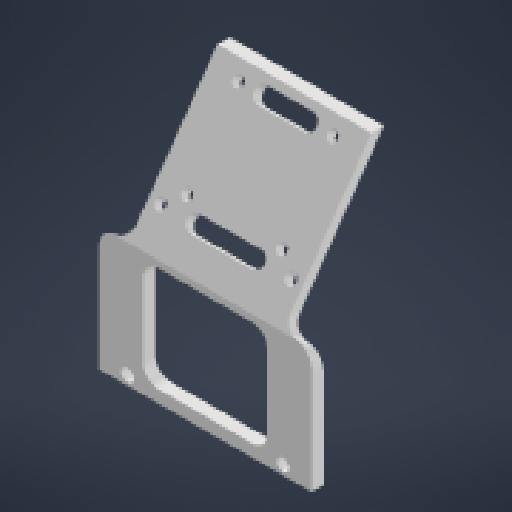
# Autodesk Inventor part: UserInterface mount
Saved by Autodesk Inventor 2023 (Build 270158000, 158)
## iProperties
Created: 2024-01-05
Part Number: UserInterface mount
Material: Generic
Document SubType Name: Modeling
Designer: nick_
Density: 1 g/cm^3
Appearance: Default
Author: nick_
Autodesk Inventor part; units mm, degrees
ref_plane "YZ Plane" through (0, 0, 0) normal (1, 0, 0) x (0, 1, 0)
ref_plane "XZ Plane" through (0, 0, 0) normal (0, 1, 0) x (-1, 0, 0)
ref_plane "XY Plane" through (0, 0, 0) normal (0, 0, 1) x (1, 0, 0)
sketch "Sketch1" plane through (0, 0, 0) normal (0, 0, 1) x (1, 0, 0)
  circle A0 centre (42.125, -15.4) radius 2 construction
  circle A1 centre (-7.875, -15.4) radius 2 construction
  line L0 (-4.825, -12.4) -> (-2.825, -14.4) construction
  line L1 (-9.825, -12.4) -> (-4.825, -12.4) construction
  arc A2 (-14.825, -7.4) -> (-9.825, -12.4) centre (-9.825, -7.4) ccw construction
  line L2 (-14.825, -7.4) -> (-14.825, 13.6) construction
  line L3 (-14.825, 13.6) -> (-15.625, 13.6) construction
  line L4 (-15.625, 13.6) -> (-15.625, 14.6) construction
  line L5 (-14.825, 15.4) -> (-15.625, 14.6) construction
  line L6 (-14.825, 15.4) -> (-14.825, 18.4) construction
  line L7 (-14.825, 18.4) -> (-17.125, 18.4) construction
  line L8 (-17.125, 18.4) -> (-17.125, -18.4) construction
  line L9 (-17.125, -18.4) -> (51.375, -18.4) construction
  line L10 (51.375, 18.4) -> (51.375, -18.4) construction
  line L11 (49.075, 18.4) -> (51.375, 18.4) construction
  line L12 (49.075, 15.4) -> (49.075, 18.4) construction
  line L13 (49.875, 14.6) -> (49.075, 15.4) construction
  line L14 (49.875, 13.6) -> (49.875, 14.6) construction
  line L15 (49.075, 13.6) -> (49.875, 13.6) construction
  line L16 (49.075, -7.4) -> (49.075, 13.6) construction
  arc A3 (44.075, -12.4) -> (49.075, -7.4) centre (44.075, -7.4) ccw construction
  line L17 (39.075, -12.4) -> (44.075, -12.4) construction
  line L18 (37.075, -14.4) -> (39.075, -12.4) construction
  line L19 (37.075, -14.4) -> (-2.825, -14.4) construction
  line L20 (-17.125, -18.4) -> (51.375, -18.4)
  line L21 (51.375, -18.4) -> (51.375, 21.449)
  line L22 (51.375, 21.449) -> (-17.125, 21.449)
  line L23 (-17.125, 21.449) -> (-17.125, -18.4)
  point P0 (0, 0)
  constraints: 8 end point, 2 collinear, 1 perpendicular, 1 point on line
extrude "Extrusion1" add sketch "Sketch1" along normal blind 4
sketch "Sketch2" plane through (51.375, -18.4, 0) normal (1, 0, 0) x (0, 0, -1)
  line L0 (0, 0) -> (0, 39.849) construction
  line L1 (0, 39.849) -> (-4, 39.849) construction
  line L2 (-4, 0) -> (-4, 39.849) construction
  line L3 (0, 0) -> (-4, 0) construction
  line L4 (-4, 39.849) -> (24.6788, 80.8066)
  line L5 (24.6788, 80.8066) -> (28.6788, 80.8066)
  line L6 (28.6788, 80.8066) -> (0, 39.849)
  line L7 (-4, 39.849) -> (0, 39.849)
  point P0 (0, 18.4)
  dimension "d2" = 55
  dimension "d5" = 50
  constraints: 8 end point, 2 equal length, 1 horizontal
  measures "d2" angle of L1 L4
  measures "d5" distance of L1.end L4.end
extrude "Extrusion2" add sketch "Sketch2" against normal up to surface (68.5 mm away)
sketch "Sketch4" plane through (-17.125, 21.449, 4) normal (0, 0.5735764, 0.819152) x (1, 0, 0)
  line L0 (22.585, 45) -> (45.915, 45) construction
  line L1 (45.915, 45) -> (45.915, 22.57) construction
  line L2 (45.915, 22.57) -> (22.585, 22.57) construction
  line L3 (22.585, 22.57) -> (22.585, 45) construction
  line L4 (68.5, 50) -> (0, 50) construction
  point P0 (17.125, -15.2757)
  point P1 (34.25, 45)
  point P2 (34.25, 50)
  dimension "d11" = 23.33
  dimension "d12" = 22.43
  dimension "d13" = 5
  constraints: 8 end point, 4 coincident, 2 midpoint, 2 parallel, 1 horizontal, 1 perpendicular, 1 vertical alignment
  measures "d11" distance of L0.start L0.end
  measures "d12" distance of L0.end L1.end
  measures "d13" distance between parallel lines of L4 L0
hole "Hole1" at (5.46, 58.3109, -21.8109) at (28.79, 58.3109, -21.8109) at (28.79, 39.9373, -8.9456) at (5.46, 39.9373, -8.9456) direction (0, -0.5735764, -0.819152) diameter 3.5 end through all
sketch "Sketch5" plane through (-17.125, 21.449, 4) normal (0, 0.5735764, 0.819152) x (1, 0, 0)
  circle A0 centre (45.915, 22.57) radius 1.75 projected
  circle A1 centre (22.585, 45) radius 1.75 projected
  circle A2 centre (45.915, 45) radius 1.75 projected
  circle A3 centre (22.585, 22.57) radius 1.75 projected
  line L0 (0, 50) -> (0, 0) projected
  line L1 (68.5, 0) -> (0, 0) projected
  line L2 (68.5, 50) -> (68.5, 0) projected
  line L3 (68.5, 50) -> (0, 50) projected
  line L4 (28.75, 45) -> (39.75, 45) construction
  line L5 (28.75, 47.5) -> (39.75, 47.5)
  line L6 (39.75, 42.5) -> (28.75, 42.5)
  arc A4 (28.75, 47.5) -> (28.75, 42.5) centre (28.75, 45) ccw
  arc A5 (39.75, 42.5) -> (39.75, 47.5) centre (39.75, 45) ccw
  point P0 (17.125, -15.2757)
  point P1 (34.25, 45)
  dimension "d25" = 23.33
  dimension "d26" = 5
  dimension "d27" = 11
  dimension "d28" = 11.665
  constraints: 8 end point, 4 point on circle, 4 tangent, 2 centre point, 1 horizontal, 1 horizontal alignment, 1 midpoint, 1 parallel
  measures "d25" distance of A2.centre A1.centre
  measures "d26" distance between parallel lines of L6 L5
  measures "d27" distance of L4.start L4.end
  measures "d28" distance of A1.centre point (34.25, 45)
extrude "Extrusion3" cut sketch "Sketch5" against normal through all contours L5 A5 L6 A4
sketch "Sketch6" plane through (-17.125, 21.449, 4) normal (0, 0.5735764, 0.819152) x (1, 0, 0)
  line L0 (24.25, 17.57) -> (44.25, 17.57) construction
  line L1 (24.25, 15.07) -> (44.25, 15.07)
  line L2 (44.25, 20.07) -> (24.25, 20.07)
  arc A0 (24.25, 20.07) -> (24.25, 15.07) centre (24.25, 17.57) ccw
  arc A1 (44.25, 15.07) -> (44.25, 20.07) centre (44.25, 17.57) ccw
  line L3 (68.5, 0) -> (0, 0) projected
  circle A2 centre (22.585, 22.57) radius 1.75 projected
  point P0 (17.125, -15.2757)
  point P1 (34.25, 17.57)
  point P2 (34.25, 0)
  dimension "d31" = 5
  dimension "d32" = 20
  dimension "d33" = 5
  constraints: 8 end point, 4 point on circle, 4 tangent, 2 centre point, 2 midpoint, 1 horizontal, 1 parallel, 1 vertical alignment
  measures "d31" distance between parallel lines of L1 L2
  measures "d32" distance of L0.start L0.end
  measures "d33" distance from line of L0 A2.centre
extrude "Extrusion4" cut sketch "Sketch6" against normal through all contours A0 L2 A1 L1
sketch "Sketch7" plane through (-17.125, 21.449, 4) normal (0, 0.5735764, 0.819152) x (1, 0, 0)
  line L0 (24.25, 20.07) -> (44.25, 20.07) projected
  line L1 (68.5, 0) -> (0, 0) projected
  point P0 (17.125, -15.2757)
  point P1 (13.25, 11.5)
  point P2 (55.25, 11.5)
  point P3 (34.25, 20.07)
  dimension "d36" = 42
  dimension "d37" = 21
  dimension "d45" = 11.5
  constraints: 1 horizontal alignment, 1 midpoint
  measures "d36" distance of point (55.25, 11.5) point (13.25, 11.5)
  measures "d37" horizontal distance of point (34.25, 20.07) point (13.25, 11.5)
  measures "d45" distance from line of L1 point (55.25, 11.5)
hole "Hole2" at (-3.875, 30.8693, -2.5961) at (38.125, 30.8693, -2.5961) direction (0, -0.5735764, -0.819152) diameter 3.5 end through all
sketch "Sketch8" plane through (-17.125, 21.449, 4) normal (0, 0.5735764, 0.819152) x (1, 0, 0)
  line L0 (0, 25.2888) -> (68.5, 25.2888) construction
  circle A0 centre (13.25, 11.5) radius 1.75 construction
  circle A1 centre (55.25, 11.5) radius 1.75 construction
  line L1 (24.25, 20.07) -> (44.25, 20.07) construction
  arc A2 (44.25, 15.07) -> (44.25, 20.07) centre (44.25, 17.57) ccw construction
  line L2 (44.25, 15.07) -> (24.25, 15.07) construction
  arc A3 (24.25, 20.07) -> (24.25, 15.07) centre (24.25, 17.57) ccw construction
  arc A4 (28.75, 47.5) -> (28.75, 42.5) centre (28.75, 45) ccw construction
  line L3 (28.75, 47.5) -> (39.75, 47.5) construction
  arc A5 (39.75, 42.5) -> (39.75, 47.5) centre (39.75, 45) ccw construction
  line L4 (39.75, 42.5) -> (28.75, 42.5) construction
  circle A6 centre (45.915, 22.57) radius 1.75 construction
  circle A7 centre (22.585, 45) radius 1.75 construction
  circle A8 centre (45.915, 45) radius 1.75 construction
  circle A9 centre (22.585, 22.57) radius 1.75 construction
  line L5 (0, 50) -> (0, 0) construction
  line L6 (68.5, 0) -> (0, 0) construction
  line L7 (68.5, 50) -> (68.5, 0) construction
  line L8 (68.5, 50) -> (0, 50) construction
  line L9 (0, 0) -> (9.5, 0)
  line L10 (9.5, 0) -> (9.5, 54)
  line L11 (9.5, 54) -> (0, 54)
  line L12 (0, 54) -> (0, 0)
  line L13 (68.5, 0) -> (59, 0)
  line L14 (59, 0) -> (59, 54)
  line L15 (59, 54) -> (68.5, 54)
  line L16 (68.5, 54) -> (68.5, 0)
  point P0 (17.125, -15.2757)
  dimension "d50" = 9.5
  dimension "d51" = 9.5
  dimension "d52" = 4
  constraints: 16 end point, 4 parallel, 2 horizontal, 2 perpendicular, 1 horizontal alignment
  measures "d50" distance of L11.end L10.end
  measures "d51" distance of L14.end L15.end
  measures "d52" distance between parallel lines of L8 L11
extrude "Extrusion5" cut sketch "Sketch8" against normal through all
fillet "Fillet1" radius 5 2 edges at (41.875, 20.0486, 2) (-7.625, 20.0486, 2)
sketch "Sketch9" plane through (0, 0, 4) normal (0, 0, 1) x (1, 0, 0)
  line L0 (-15.875, 15.26) -> (50.125, 15.26) construction
  line L1 (50.125, 15.26) -> (50.125, 13.6) construction
  line L2 (-15.875, 13.6) -> (50.125, 13.6) construction
  line L3 (-15.875, 15.26) -> (-15.875, 13.6) construction
  line L4 (-2.825, -14.4) -> (37.075, -14.4) construction
  line L5 (37.075, -14.4) -> (-2.825, -14.4)
  line L6 (-2.825, -14.4) -> (-2.825, 19.26)
  line L7 (-2.825, 19.26) -> (37.075, 19.26)
  line L8 (37.075, 19.26) -> (37.075, -14.4)
  point P0 (0, 0)
  dimension "d54" = 4
  constraints: 8 end point, 2 parallel, 1 horizontal, 1 perpendicular, 1 point on line
  measures "d54" distance between parallel lines of L0 L7
extrude "Extrusion6" cut sketch "Sketch9" against normal through all
fillet "Fillet2" radius 5 6 edges at (-2.825, 19.26, 2) (37.075, 19.26, 2) (37.075, -14.4, 2) (-2.825, -14.4, 2) (51.375, 20.0486, 2) (-17.125, 20.0486, 2)
sketch "Sketch10" plane through (0, 0, 4) normal (0, 0, 1) x (1, 0, 0)
  circle A0 centre (-7.875, -15.4) radius 2 construction
  circle A1 centre (42.125, -15.4) radius 2 construction
  point P0 (0, 0)
  constraints: 2 coincident
hole "Hole3" at (-7.875, -15.4, 4) at (42.125, -15.4, 4) direction (0, 0, -1) diameter 4 end through all
fillet "Fillet3" radius 5 1 edges at (17.125, 21.449, 0)
equation "\"d28\" = 0.5 * d25"
equation "\"d37\" = 0.5 * d36"
equation "\"d51\" = d50"
body "Solid1"
